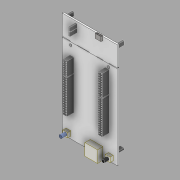
# Autodesk Inventor part: nucleo_746zg
Saved by Autodesk Inventor 2021 (Build 250183000, 183)
## iProperties
Created: 2022-05-17
Part Number: nucleo_746zg
Material: Generic
Document SubType Name: Modeling
Designer: agnpi
Density: 1 g/cm^3
Appearance: Default
Author: agnpi
Autodesk Inventor part; units mm, degrees
ref_plane "YZ Plane" through (0, 0, 0) normal (1, 0, 0) x (0, 1, 0)
ref_plane "XZ Plane" through (0, 0, 0) normal (0, 1, 0) x (-1, 0, 0)
ref_plane "XY Plane" through (0, 0, 0) normal (0, 0, 1) x (1, 0, 0)
sketch "Sketch1" plane through (0, 0, 0) normal (0, 0, 1) x (1, 0, 0)
  line L0 (-49, 0) -> (49, 0) projected
  line L1 (0, -74.9) -> (0, 74.9) projected
  line L2 (-35, 53.5) -> (35, 53.5)
  line L3 (35, 53.5) -> (35, -53.5)
  line L4 (35, -53.5) -> (-35, -53.5)
  line L5 (-35, -53.5) -> (-35, 53.5)
  line L6 (-35, 53.5) -> (35, -53.5) construction
  line L7 (35, 53.5) -> (-35, -53.5) construction
  point P0 (0, 0)
  dimension "d0" = 107
  dimension "d1" = 70
  constraints: 12 end point, 2 midpoint, 2 parallel, 1 horizontal, 1 perpendicular
  measures "d0" distance of L2.end L3.end
  measures "d1" distance between parallel lines of L3 L5
extrude "Extrusion1" add sketch "Sketch1" along normal mid plane 2
sketch "Sketch2" plane through (0, 0, 1) normal (0, 0, 1) x (1, 0, 0)
  line L0 (20, 47.5) -> (25, 47.5)
  line L1 (25, -22.5) -> (20, -22.5)
  line L2 (20, 47.5) -> (25, -22.5) construction
  line L3 (25, 47.5) -> (20, -22.5) construction
  line L4 (20, 20.5) -> (25, 20.5)
  line L5 (20, 19.5) -> (25, 19.5)
  line L6 (25, 47.5) -> (25, 20.5)
  line L7 (25, 19.5) -> (25, -22.5)
  line L8 (20, -22.5) -> (20, 19.5)
  line L9 (20, 20.5) -> (20, 47.5)
  line L10 (35, -53.5) -> (35, 53.5) projected
  line L11 (35, 53.5) -> (-35, 53.5) projected
  line L12 (-25, 38.5) -> (-20, 38.5)
  line L13 (-20, 38.5) -> (-20, 21.049)
  line L14 (-20, 21.049) -> (-25, 21.049)
  line L15 (-25, 21.049) -> (-25, 38.5)
  line L16 (-25, 38.5) -> (-20, 21.049) construction
  line L17 (-20, 38.5) -> (-25, 21.049) construction
  line L18 (-25, 20.049) -> (-20, 20.049)
  line L19 (-20, 20.049) -> (-20, -22.5)
  line L20 (-20, -22.5) -> (-25, -22.5)
  line L21 (-25, -22.5) -> (-25, 20.049)
  line L22 (-25, 20.049) -> (-20, -22.5) construction
  line L23 (-20, 20.049) -> (-25, -22.5) construction
  line L24 (-35, 53.5) -> (-35, -53.5) projected
  line L25 (-35, -53.5) -> (35, -53.5) projected
  point P0 (0, 0)
  point P1 (22.5, 12.5)
  point P2 (-22.5, 29.7745)
  point P3 (-22.5, -1.2255)
  dimension "d4" = 70
  dimension "d5" = 27
  dimension "d6" = 1
  dimension "d7" = 5
  dimension "d8" = 5
  dimension "d9" = 10
  dimension "d10" = 10
  dimension "d11" = 6
  dimension "d12" = 10
  dimension "d13" = 10
  dimension "d14" = 5
  dimension "d15" = 5
  dimension "d112" = 17.451
  dimension "d113" = 31
  dimension "d114" = 61
  dimension "d115" = 1
  constraints: 44 end point, 9 parallel, 8 perpendicular, 6 midpoint, 3 horizontal
  measures "d4" distance between parallel lines of L1 L0
  measures "d5" distance between parallel lines of L0 L4
  measures "d6" distance between parallel lines of L5 L4
  measures "d7" distance between parallel lines of L7 L8
  measures "d8" distance between parallel lines of L6 L9
  measures "d9" distance between parallel lines of L10 L6
  measures "d10" distance between parallel lines of L10 L7
  measures "d11" distance between parallel lines of L11 L0
  measures "d12" distance between parallel lines of L24 L15
  measures "d13" distance between parallel lines of L24 L21
  measures "d14" distance between parallel lines of L13 L15
  measures "d15" distance between parallel lines of L19 L21
  measures "d112" distance of L12.end L13.end
  measures "d113" distance between parallel lines of L25 L20
  measures "d114" distance of L12.start L20.end
  measures "d115" distance between parallel lines of L14 L18
extrude "Extrusion2" add sketch "Sketch2" along normal blind 9 separate body contours L0 L6 L4 L9 | L1 L8 L5 L7 | L12 L13 L14 L15 | L18 L19 L20 L21
sketch "Sketch3" plane through (0, 0, 1) normal (0, 0, 1) x (1, 0, 0)
  line L0 (35, 53.5) -> (-35, 53.5) projected
  line L1 (35, -53.5) -> (35, 53.5) projected
  point P0 (0, 0)
  point P1 (24.13, 49.8)
  point P2 (-24.13, 49.8)
  dimension "d27" = 48.26
  dimension "d28" = 3.7
  dimension "d29" = 3.7
  dimension "d30" = 10.87
  measures "d27" distance of point (24.13, 49.8) point (-24.13, 49.8)
  measures "d28" distance from line of L0 point (-24.13, 49.8)
  measures "d29" distance from line of L0 point (24.13, 49.8)
  measures "d30" distance from line of L1 point (24.13, 49.8)
hole "Hole1" at (24.13, 49.8, 1) at (-24.13, 49.8, 1) direction (0, 0, -1) diameter 3 end through all bodies 1
sketch "Sketch4" plane through (0, 0, 1) normal (0, 0, 1) x (1, 0, 0)
  line L0 (1, -41.5) -> (17, -41.5)
  line L1 (17, -41.5) -> (17, -56.5)
  line L2 (17, -56.5) -> (1, -56.5)
  line L3 (1, -56.5) -> (1, -41.5)
  line L4 (1, -41.5) -> (17, -56.5) construction
  line L5 (17, -41.5) -> (1, -56.5) construction
  line L6 (35, -53.5) -> (35, 53.5) projected
  line L7 (-35, -53.5) -> (35, -53.5) projected
  point P0 (0, 0)
  point P1 (9, -49)
  dimension "d31" = 16
  dimension "d32" = 15
  dimension "d33" = 18
  dimension "d34" = 3
  constraints: 12 end point, 2 midpoint, 2 parallel, 1 horizontal, 1 perpendicular
  measures "d31" distance between parallel lines of L1 L3
  measures "d32" distance between parallel lines of L2 L0
  measures "d33" distance between parallel lines of L6 L1
  measures "d34" distance between parallel lines of L7 L2
extrude "Extrusion3" add sketch "Sketch4" along normal blind 7 separate body
sketch "Sketch5" plane through (0, 0, 1) normal (0, 0, -1) x (-1, 0, 0)
  point P0 (0, 0)
sketch "Sketch7" plane through (-35, -53.5, 1) normal (0, -1, 0) x (1, 0, 0)
  line L0 (36, 0) -> (36, 7) projected
  line L1 (36, 0) -> (52, 0)
  line L2 (52, 0) -> (52, -3.1591)
  line L3 (52, -3.1591) -> (36, -3.1591)
  line L4 (36, -3.1591) -> (36, 0)
  point P0 (35, -1)
  constraints: 8 end point, 2 parallel, 1 horizontal, 1 perpendicular
extrude "Extrusion4" add sketch "Sketch7" along normal blind 3 separate body
sketch "Sketch8" plane through (0, 0, -1) normal (0, 0, -1) x (-1, 0, 0)
  line L0 (-1, -41.5) -> (-1, -56.5) projected
  line L1 (-17, -56.5) -> (-17, -41.5) projected
  line L2 (-1, -53.5) -> (-17, -53.5)
  line L3 (-17, -53.5) -> (-17, -45.5)
  line L4 (-17, -45.5) -> (-1, -45.5)
  line L5 (-1, -45.5) -> (-1, -53.5)
  line L6 (-1, -56.5) -> (-17, -56.5) projected
  point P0 (0, 0)
  point P1 (-1, -45.5)
  dimension "d39" = 11
  constraints: 8 end point, 3 point on line, 2 parallel, 1 horizontal, 1 perpendicular
  measures "d39" distance between parallel lines of L4 L6
extrude "Extrusion5" add sketch "Sketch8" along normal blind 1 separate body contours L0 L2 L1 L4
sketch "Sketch10" plane through (0, 0, -1) normal (0, 0, -1) x (-1, 0, 0)
  line L0 (-25, 20.5) -> (-25, 47.5) projected
  line L1 (-20, 47.5) -> (-20, 20.5) projected
  line L2 (-25, 47.5) -> (-20, 47.5)
  line L3 (-20, 47.5) -> (-20, 20.5)
  line L4 (-20, 20.5) -> (-25, 20.5)
  line L5 (-25, 20.5) -> (-25, 47.5)
  line L6 (-25, 19.5) -> (-20, 19.5) projected
  line L7 (-20, -22.5) -> (-25, -22.5) projected
  line L8 (-25, 19.5) -> (-20, 19.5)
  line L9 (-20, 19.5) -> (-20, -22.5)
  line L10 (-20, -22.5) -> (-25, -22.5)
  line L11 (-25, -22.5) -> (-25, 19.5)
  line L12 (20, 21.049) -> (20, 38.5) projected
  line L13 (25, 38.5) -> (25, 21.049) projected
  line L14 (20, 38.5) -> (25, 38.5)
  line L15 (25, 38.5) -> (25, 21.049)
  line L16 (25, 21.049) -> (20, 21.049)
  line L17 (20, 21.049) -> (20, 38.5)
  line L18 (20, 20.049) -> (25, 20.049) projected
  line L19 (25, -22.5) -> (20, -22.5) projected
  line L20 (20, 20.049) -> (25, 20.049)
  line L21 (25, 20.049) -> (25, -22.5)
  line L22 (25, -22.5) -> (20, -22.5)
  line L23 (20, -22.5) -> (20, 20.049)
  point P0 (0, 0)
  point P1 (25, 20.049)
  point P2 (25, 38.5)
  constraints: 32 end point, 8 parallel, 4 horizontal, 4 perpendicular
extrude "Extrusion6" add sketch "Sketch10" along normal blind 7.5 separate body
sketch "Sketch11" plane through (0, 0, 1) normal (0, 0, 1) x (1, 0, 0)
  line L0 (-30, -44.5) -> (-24, -44.5)
  line L1 (-24, -44.5) -> (-24, -50.5)
  line L2 (-24, -50.5) -> (-30, -50.5)
  line L3 (-30, -50.5) -> (-30, -44.5)
  line L4 (24, -44.5) -> (30, -44.5)
  line L5 (30, -44.5) -> (30, -50.5)
  line L6 (30, -50.5) -> (24, -50.5)
  line L7 (24, -50.5) -> (24, -44.5)
  line L8 (-35, -53.5) -> (35, -53.5) projected
  line L9 (35, -53.5) -> (35, 53.5) projected
  line L10 (-35, 53.5) -> (-35, -53.5) projected
  point P0 (0, 0)
  dimension "d59" = 3
  dimension "d60" = 3
  dimension "d61" = 6
  dimension "d62" = 6
  dimension "d63" = 6
  dimension "d64" = 6
  dimension "d65" = 5
  dimension "d66" = 5
  constraints: 16 end point, 4 parallel, 2 horizontal, 2 perpendicular
  measures "d59" distance between parallel lines of L8 L2
  measures "d60" distance between parallel lines of L8 L6
  measures "d61" distance between parallel lines of L6 L4
  measures "d62" distance between parallel lines of L5 L7
  measures "d63" distance of L0.start L0.end
  measures "d64" distance of L0.end L1.end
  measures "d65" distance between parallel lines of L9 L5
  measures "d66" distance between parallel lines of L10 L3
extrude "Extrusion7" add sketch "Sketch11" along normal blind 4 separate body
sketch "Sketch12" plane through (0, 0, 5) normal (0, 0, 1) x (1, 0, 0)
  circle A0 centre (-27, -47.5) radius 2
  circle A1 centre (27, -47.5) radius 2
  line L0 (30, -44.5) -> (24, -44.5) projected
  line L1 (24, -44.5) -> (24, -50.5) projected
  line L2 (-24, -44.5) -> (-30, -44.5) projected
  line L3 (-24, -50.5) -> (-24, -44.5) projected
  point P0 (0, 0)
  dimension "d69" = 4
  dimension "d70" = 4
  dimension "d71" = 3
  dimension "d72" = 3
  dimension "d73" = 3
  dimension "d74" = 3
  constraints: 2 centre point
  measures "d69" diameter of A0
  measures "d70" diameter of A1
  measures "d71" distance from line of L0 A1.centre
  measures "d72" distance from line of L1 A1.centre
  measures "d73" distance from line of L2 A0.centre
  measures "d74" distance from line of L3 A0.centre
extrude "Extrusion8" add sketch "Sketch12" along normal blind 6 separate body contours A0
extrude "Extrusion9" add sketch "Sketch12" along normal blind 6 separate body contours A1
sketch "Sketch13" plane through (-35, 53.5, 1) normal (0, 1, 0) x (1, 0, 0)
  line L0 (0, 2) -> (0, 0) projected
  line L1 (70, 0) -> (0, 0) projected
  line L2 (0, 2) -> (70, 2)
  line L3 (70, 2) -> (70, 0)
  line L4 (70, 0) -> (0, 0)
  line L5 (0, 0) -> (0, 2)
  point P0 (35, 1)
  constraints: 8 end point, 2 parallel, 1 horizontal, 1 perpendicular
extrude "Extrusion10" add sketch "Sketch13" along normal blind 26.34 separate body
sketch "Sketch14" plane through (35, 53.5, -1) normal (0, 0, -1) x (-1, 0, 0)
  line L0 (2, 24.34) -> (4, 24.34)
  line L1 (4, 24.34) -> (4, 19.34)
  line L2 (4, 19.34) -> (2, 19.34)
  line L3 (2, 19.34) -> (2, 24.34)
  line L4 (66, 24.34) -> (68, 24.34)
  line L5 (68, 24.34) -> (68, 19.34)
  line L6 (68, 19.34) -> (66, 19.34)
  line L7 (66, 19.34) -> (66, 24.34)
  line L8 (70, 0) -> (70, 26.34) projected
  line L9 (0, 0) -> (0, 26.34) projected
  line L10 (0, 26.34) -> (70, 26.34) projected
  point P0 (35, -53.5)
  dimension "d81" = 5
  dimension "d82" = 2
  dimension "d83" = 2
  dimension "d84" = 2
  dimension "d85" = 2
  dimension "d86" = 2
  constraints: 16 end point, 4 parallel, 2 horizontal, 2 perpendicular, 2 point on line
  measures "d81" distance between parallel lines of L6 L4
  measures "d82" distance between parallel lines of L5 L7
  measures "d83" distance of L1.end L2.end
  measures "d84" distance between parallel lines of L8 L5
  measures "d85" distance between parallel lines of L9 L3
  measures "d86" distance between parallel lines of L10 L0
extrude "Extrusion11" add sketch "Sketch14" along normal blind 9 separate body
sketch "Sketch15" plane through (0, 0, -1) normal (0, 0, -1) x (-1, 0, 0)
  line L0 (-33, -40.5) -> (-28, -40.5)
  line L1 (-28, -40.5) -> (-28, -42.5)
  line L2 (-28, -42.5) -> (-33, -42.5)
  line L3 (-33, -42.5) -> (-33, -40.5)
  line L4 (28, -40.5) -> (33, -40.5)
  line L5 (33, -40.5) -> (33, -42.5)
  line L6 (33, -42.5) -> (28, -42.5)
  line L7 (28, -42.5) -> (28, -40.5)
  line L8 (-35, 53.5) -> (-35, -53.5) projected
  line L9 (35, -53.5) -> (35, 53.5) projected
  line L10 (-35, -53.5) -> (35, -53.5) projected
  point P0 (0, 0)
  dimension "d89" = 5
  dimension "d90" = 5
  dimension "d91" = 2
  dimension "d92" = 2
  dimension "d93" = 2
  dimension "d94" = 11
  constraints: 16 end point, 4 parallel, 2 horizontal, 2 perpendicular, 2 point on line
  measures "d89" distance of L0.end L0.start
  measures "d90" distance of L4.end L4.start
  measures "d91" distance from line of L5.end L4
  measures "d92" distance from line of L8 L0.start
  measures "d93" distance from line of L9 L4.end
  measures "d94" distance between parallel lines of L10 L2
extrude "Extrusion12" add sketch "Sketch15" along normal blind 9 separate body
sketch "Sketch16" plane through (-35, 53.5, 1) normal (0, 0, 1) x (1, 0, 0)
  line L0 (44.5, 27.34) -> (52, 27.34)
  line L1 (52, 27.34) -> (52, 21.84)
  line L2 (52, 21.84) -> (44.5, 21.84)
  line L3 (44.5, 21.84) -> (44.5, 27.34)
  line L4 (70, 0) -> (70, 26.34) projected
  line L5 (0, 26.34) -> (70, 26.34) projected
  point P0 (35, -53.5)
  dimension "d97" = 7.5
  dimension "d98" = 5.5
  dimension "d99" = 18
  dimension "d100" = 4.5
  constraints: 8 end point, 2 parallel, 1 horizontal, 1 perpendicular
  measures "d97" distance between parallel lines of L1 L3
  measures "d98" distance between parallel lines of L2 L0
  measures "d99" distance between parallel lines of L4 L1
  measures "d100" distance between parallel lines of L5 L2
extrude "Extrusion13" add sketch "Sketch16" along normal blind 2.5 separate body
sketch "Sketch17" plane through (-35, 53.5, 1) normal (0, 0, 1) x (1, 0, 0)
  line L0 (17, 24.34) -> (19, 24.34)
  line L1 (19, 24.34) -> (19, 19.34)
  line L2 (19, 19.34) -> (17, 19.34)
  line L3 (17, 19.34) -> (17, 24.34)
  line L4 (17, 19.04) -> (19, 19.04)
  line L5 (19, 19.04) -> (19, 14.04)
  line L6 (19, 14.04) -> (17, 14.04)
  line L7 (17, 14.04) -> (17, 19.04)
  line L8 (0, 26.34) -> (70, 26.34) projected
  line L9 (0, 0) -> (0, 26.34) projected
  point P0 (35, -53.5)
  dimension "d103" = 2
  dimension "d104" = 5
  dimension "d105" = 5
  dimension "d106" = 0.3
  dimension "d107" = 2
  dimension "d108" = 17
  constraints: 16 end point, 4 parallel, 2 horizontal, 2 perpendicular, 2 point on line
  measures "d103" distance between parallel lines of L1 L3
  measures "d104" distance between parallel lines of L6 L4
  measures "d105" distance between parallel lines of L2 L0
  measures "d106" distance between parallel lines of L4 L2
  measures "d107" distance between parallel lines of L8 L0
  measures "d108" distance between parallel lines of L9 L3
extrude "Extrusion14" add sketch "Sketch17" along normal blind 9 separate body
sketch "Sketch18" plane through (0, 0, 10) normal (0, 0, 1) x (1, 0, 0)
  circle A0 centre (-24, 36.8113) radius 0.5
  circle A1 centre (-21, 36.8113) radius 0.5
  line L0 (-25, 38.5) -> (-25, 21.049) projected
  line L1 (-20, 21.049) -> (-20, 38.5) projected
  circle A2 centre (-24, 34.8113) radius 0.5
  circle A3 centre (-21, 34.8113) radius 0.5
  circle A4 centre (-24, 32.8113) radius 0.5
  circle A5 centre (-21, 32.8113) radius 0.5
  circle A6 centre (-24, 30.8113) radius 0.5
  circle A7 centre (-21, 30.8113) radius 0.5
  circle A8 centre (-24, 28.8113) radius 0.5
  circle A9 centre (-21, 28.8113) radius 0.5
  circle A10 centre (-24, 26.8113) radius 0.5
  circle A11 centre (-21, 26.8113) radius 0.5
  circle A12 centre (-24, 24.8113) radius 0.5
  circle A13 centre (-21, 24.8113) radius 0.5
  circle A14 centre (-24, 22.8113) radius 0.5
  circle A15 centre (-21, 22.8113) radius 0.5
  line L2 (-25, 21.049) -> (-20, 21.049) projected
  point P0 (0, 0)
  dimension "d116" = 1
  dimension "d117" = 1
  dimension "d118" = 1
  dimension "d119" = 1
  dimension "d120" = 3
  dimension "d127" = 2
  dimension "d129" = 1.7623
  constraints: 16 centre point, 1 vertical, 28 other
  measures "d116" diameter of A0
  measures "d117" diameter of A1
  measures "d118" distance from line of L0 A0.centre
  measures "d119" distance from line of L1 A1.centre
  measures "d120" distance of A1.centre A0.centre
  measures "d127" distance of A0.centre A2.centre
  measures "d129" distance from line of L2 A15.centre
extrude "Extrusion15" cut sketch "Sketch18" against normal blind 4 bodies 2
sketch "Sketch19" plane through (0, 0, 10) normal (0, 0, 1) x (1, 0, 0)
  circle A0 centre (-24.0412, 18.1489) radius 0.5
  circle A1 centre (-21.0412, 18.1489) radius 0.5
  line L0 (-20, 20.049) -> (-25, 20.049) projected
  line L1 (-20, -22.5) -> (-20, 20.049) projected
  point P0 (0, 0)
  dimension "d132" = 1
  dimension "d133" = 1
  dimension "d134" = 3
  dimension "d135" = 1.9001
  dimension "d136" = 1.9001
  dimension "d137" = 1.0412
  constraints: 2 centre point
  measures "d132" diameter of A0
  measures "d133" diameter of A1
  measures "d134" distance of A1.centre A0.centre
  measures "d135" distance from line of L0 A0.centre
  measures "d136" distance from line of L0 A1.centre
  measures "d137" distance from line of L1 A1.centre
extrude "Extrusion16" cut sketch "Sketch19" against normal blind 4 bodies 2
pattern_linear "Rectangular Pattern1" count 15 spacing 2.7 along (0, -1, 0) of "Extrusion16" bodies 2
sketch "Sketch20" plane through (0, 0, 10) normal (0, 0, 1) x (1, 0, 0)
  circle A0 centre (21, 18) radius 0.5
  circle A1 centre (24, 18) radius 0.5
  line L0 (25, 19.5) -> (20, 19.5) projected
  line L1 (20, 19.5) -> (20, -22.5) projected
  point P0 (0, 0)
  dimension "d143" = 1
  dimension "d144" = 1
  dimension "d145" = 3
  dimension "d146" = 1.5
  dimension "d147" = 1.5
  dimension "d148" = 1
  constraints: 2 centre point
  measures "d143" diameter of A0
  measures "d144" diameter of A1
  measures "d145" distance of A1.centre A0.centre
  measures "d146" distance from line of L0 A0.centre
  measures "d147" distance from line of L0 A1.centre
  measures "d148" distance from line of L1 A0.centre
extrude "Extrusion17" cut sketch "Sketch20" against normal blind 4 bodies 2
pattern_linear "Rectangular Pattern2" count 17 spacing 2.4 along (0, -1, 0) of "Extrusion17" bodies 2
sketch "Sketch21" plane through (0, 0, 10) normal (0, 0, 1) x (1, 0, 0)
  circle A0 centre (21, 46.5) radius 0.5
  circle A1 centre (24, 46.5) radius 0.5
  line L0 (25, 20.5) -> (25, 47.5) projected
  line L1 (20, 47.5) -> (20, 20.5) projected
  line L2 (25, 47.5) -> (20, 47.5) projected
  point P0 (0, 0)
  dimension "d154" = 1
  dimension "d155" = 1
  dimension "d156" = 3
  dimension "d157" = 1
  dimension "d158" = 1
  dimension "d159" = 1
  constraints: 2 centre point
  measures "d154" diameter of A0
  measures "d155" diameter of A1
  measures "d156" distance of A1.centre A0.centre
  measures "d157" distance from line of L0 A1.centre
  measures "d158" distance from line of L1 A0.centre
  measures "d159" distance from line of L2 A0.centre
extrude "Extrusion18" cut sketch "Sketch21" against normal blind 4 bodies 2
pattern_linear "Rectangular Pattern3" count 10 spacing 2.7 along (0, -1, 0) of "Extrusion18" bodies 2
sketch "Sketch22" plane through (9.5, 80.84, 1) normal (0, 1, 0) x (1, 0, 0)
  line L0 (1.25, -0.75) -> (6.25, -0.75)
  line L1 (6.25, -0.75) -> (6.25, -1.75)
  line L2 (6.25, -1.75) -> (1.25, -1.75)
  line L3 (1.25, -1.75) -> (1.25, -0.75)
  line L4 (7.5, 0) -> (7.5, -2.5) projected
  line L5 (7.5, -2.5) -> (0, -2.5) projected
  point P0 (-9.5, 1)
  dimension "d165" = 5
  dimension "d166" = 1.25
  dimension "d167" = 1
  dimension "d168" = 0.75
  constraints: 8 end point, 2 parallel, 1 horizontal, 1 perpendicular
  measures "d165" distance of L0.end L0.start
  measures "d166" distance from line of L4 L1.end
  measures "d167" distance between parallel lines of L2 L0
  measures "d168" distance between parallel lines of L5 L2
extrude "Extrusion19" cut sketch "Sketch22" against normal blind 2 bodies 13
sketch "Sketch23" plane through (-35, 53.5, 1) normal (0, 0, 1) x (1, 0, 0)
  line L0 (0, 0) -> (0, -107) projected
  line L1 (0, 0) -> (9.6, 0) construction
  line L2 (70, 0) -> (0, 0) projected
  line L3 (0, -0.75) -> (9.6, -0.75)
  line L4 (9.6, 0.75) -> (0, 0.75)
  arc A0 (9.6, -0.75) -> (9.6, 0.75) centre (9.6, 0) ccw
  line L5 (70, -0.75) -> (60.4, -0.75)
  line L6 (60.4, 0.75) -> (70, 0.75)
  arc A1 (70, -0.75) -> (70, 0.75) centre (70, 0) ccw
  arc A2 (60.4, 0.75) -> (60.4, -0.75) centre (60.4, 0) ccw
  line L7 (0, 26.34) -> (70, 26.34) projected
  line L8 (44.4346, 0) -> (51.4346, 0) construction
  line L9 (44.4346, -0.5) -> (51.4346, -0.5)
  line L10 (51.4346, 0.5) -> (44.4346, 0.5)
  arc A3 (44.4346, 0.5) -> (44.4346, -0.5) centre (44.4346, 0) ccw
  arc A4 (51.4346, -0.5) -> (51.4346, 0.5) centre (51.4346, 0) ccw
  line L11 (20.0329, 0) -> (34.0329, 0) construction
  line L12 (20.0329, -0.5) -> (34.0329, -0.5)
  line L13 (34.0329, 0.5) -> (20.0329, 0.5)
  arc A5 (20.0329, 0.5) -> (20.0329, -0.5) centre (20.0329, 0) ccw
  arc A6 (34.0329, -0.5) -> (34.0329, 0.5) centre (34.0329, 0) ccw
  line L14 (0, -0.75) -> (0, 0.75)
  point P0 (35, -53.5)
  point P1 (4.8, 0)
  point P2 (65.2, 0)
  point P3 (47.9346, 0)
  point P4 (27.0329, 0)
  point P5 (51.9346, 0)
  point P6 (43.9346, 0)
  point P7 (10.35, 0)
  dimension "d171" = 1.5
  dimension "d173" = 11.1
  dimension "d174" = 0.75
  dimension "d175" = 0.75
  dimension "d176" = 9.6
  dimension "d177" = 9.6
  dimension "d178" = 4.8
  dimension "d179" = 25.59
  dimension "d180" = 27.09
  dimension "d181" = 0
  dimension "d182" = 1
  dimension "d183" = 8
  dimension "d184" = 51.4346
  dimension "d185" = 1
  dimension "d186" = 15
  dimension "d187" = 9.4018
  dimension "d200" = 90
  dimension "d201" = 0
  dimension "d202" = 0
  dimension "d203" = 51.9346
  dimension "d204" = 0
  dimension "d205" = 43.9346
  dimension "d206" = 0
  dimension "d207" = 10.35
  dimension "d208" = 9.6
  dimension "d209" = 0
  dimension "d210" = 0
  constraints: 30 end point, 14 point on circle, 10 tangent, 7 centre point, 5 point on line, 3 midpoint, 3 parallel, 1 vertical
  measures "d171" diameter of A0
  measures "d174" radius of A1
  measures "d175" radius of A2
  measures "d176" distance of L5.start L5.end
  measures "d177" distance of L6.start L6.end
  measures "d178" distance of A2.centre point (65.2, 0)
  measures "d179" distance between parallel lines of L7 L6
  measures "d180" distance from line of L7.end L5
  measures "d181" distance from line of point (65.2, 0) L2
  measures "d182" diameter of A4
  measures "d184" distance from line of L10.start L0
  measures "d185" diameter of A6
  measures "d200" angle of L4 L0
  measures "d201" distance between parallel lines of L14 L0
  measures "d202" distance from line of point (51.935, 0) L2
  measures "d203" distance from line of point (51.935, 0) L0
  measures "d204" distance from line of point (43.935, 0) L2
  measures "d205" distance from line of point (43.935, 0) L0
  measures "d206" distance from line of point (10.35, 0) L2
  measures "d207" distance from line of point (10.35, 0) L0
  measures "d208" distance from line of L4.start L0
  measures "d209" distance from line of point (0, 0) L2
  measures "d210" distance from line of point (0, 0) L0
extrude "Extrusion23" cut sketch "Sketch23" against normal through all contours L2 A0 L3 L0 | L14 L4 A0 L2 bodies 10
extrude "Extrusion24" cut sketch "Sketch23" against normal through all contours A2 L6 A1 L5 | A3 L10 A4 L2 | L2 A4 L9 A3 | A5 L13 A6 L2 | L2 A6 L12 A5 bodies 10
body "Solid1"
body "Solid2"
body "Solid3"
body "Solid4"
body "Solid5"
body "Solid6"
body "Solid7"
body "Solid8"
body "Solid9"
body "Solid10"
body "Solid11"
body "Solid12"
body "Solid13"
body "Solid14"
